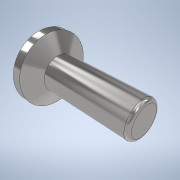
# Autodesk Inventor part: Гвоздик 4х12 мм
Saved by Autodesk Inventor 2021.1 (Build 251245010, 245A)
## iProperties
Created: 2026-05-20
Part Number: Гвоздик 4х12 мм
Material: Типовые
Document SubType Name: Modeling
Designer: Андрей Тарасов
Density: 1 g/cm^3
Appearance: По умолчанию
Author: Андрей Тарасов
Autodesk Inventor part; units mm, degrees
ref_plane "YZ Plane" through (0, 0, 0) normal (1, 0, 0) x (0, 1, 0)
ref_plane "XZ Plane" through (0, 0, 0) normal (0, 1, 0) x (-1, 0, 0)
ref_plane "XY Plane" through (0, 0, 0) normal (0, 0, 1) x (1, 0, 0)
sketch "Эскиз1" plane through (0, 0, 0) normal (0, 0, 1) x (1, 0, 0)
  line L0 (0, 0) -> (0, 4)
  line L1 (0, 4) -> (1, 4)
  line L2 (1, 4) -> (2, 2)
  line L3 (2, 2) -> (11.6, 2)
  line L4 (12, 1.6) -> (12, 0)
  line L5 (12, 0) -> (0, 0)
  arc A0 (12, 1.6) -> (11.6, 2) centre (11.6, 1.6) ccw
  point P0 (12, 2)
  dimension "d0" = 4
  dimension "d1" = 1
  dimension "d2" = 2
  dimension "d3" = 2
  dimension "d7" = 12
  dimension "d9" = 0.4
  constraints: 12 end point, 2 perpendicular, 2 point on circle, 2 point on line, 2 tangent, 2 vertical, 1 centre point
  measures "d0" distance of L0.start L0.end
  measures "d1" distance of L0.end L1.end
  measures "d2" distance from line of L0 L2.end
  measures "d3" distance between parallel lines of L5 L3
  measures "d7" distance of L4.end L0.start
  measures "d9" radius of A0
revolve "Вращение1" add sketch "Эскиз1" angle 360 about axis through (12, 0, 0) along (-1, 0, 0)
